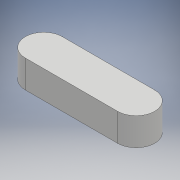
# Autodesk Inventor part: Chaveta- Tren 1
Saved by Autodesk Inventor 2018 (Build 220112000, 112)
## iProperties
Created: 2017-09-04
Part Number: Chaveta- Tren 1
Material: Genérico
Document SubType Name: Modeling
Designer: Alumno
Density: 1 g/cm^3
Appearance: Valor por defecto
Author: Alumno
Autodesk Inventor part; units mm, degrees
ref_plane "YZ Plane" through (0, 0, 0) normal (1, 0, 0) x (0, 1, 0)
ref_plane "XZ Plane" through (0, 0, 0) normal (0, 1, 0) x (-1, 0, 0)
ref_plane "XY Plane" through (0, 0, 0) normal (0, 0, 1) x (1, 0, 0)
sketch "Boceto1" plane through (0, 0, 0) normal (0, 0, 1) x (1, 0, 0)
  line L0 (10, -1.8375) -> (-10, -1.8375)
  line L1 (-10, 6.1625) -> (10, 6.1625)
  arc A0 (-10, 6.1625) -> (-10, -1.8375) centre (-10, 2.1625) ccw
  arc A1 (10, -1.8375) -> (10, 6.1625) centre (10, 2.1625) ccw
  point P0 (-0.5, 2.1625)
  point P1 (-14, 2.1625)
  dimension "d25" = 8
  dimension "d26" = 20
  constraints: 5 point on circle, 4 end point, 2 centre point, 2 tangent, 1 horizontal, 1 parallel
  measures "d25" distance between parallel lines of L0 L1
  measures "d26" distance of A1.centre A0.centre
extrude "Extrusión2" add sketch "Boceto1" along normal blind 6
